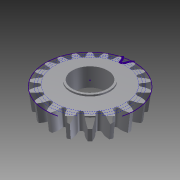
# Autodesk Inventor part: Z20
Saved by Autodesk Inventor 2014 (Build 180170000, 170)
## iProperties
Created: 2013-05-24
Part Number: Z20
Material: Generic
Document SubType Name: Modeling
Designer: hartmann
Density: 1 g/cm^3
Appearance: Default
Mass: 0.0697017 g
Surface Area: 1.89234 cm^2
Volume: 0.0697017 cm^3
Author: hartmann
Autodesk Inventor part; units mm, degrees
ref_plane "YZ Plane" through (0, 0, 0) normal (1, 0, 0) x (0, 1, 0)
ref_plane "XZ Plane" through (0, 0, 0) normal (0, 1, 0) x (-1, 0, 0)
ref_plane "XY Plane" through (0, 0, 0) normal (0, 0, 1) x (1, 0, 0)
sketch "Sketch1" plane through (0, 0, 0) normal (0, 0, 1) x (1, 0, 0)
  spline S0 degree 3 poles (-0.5498, 4.3643) (-0.5222, 4.3285) (-0.4672, 4.2569) (-0.3937, 4.1428) (-0.3394, 4.0438) (-0.3016, 3.9617) (-0.2765, 3.8987) (-0.2553, 3.8344) (-0.2398, 3.7683) (-0.2337, 3.7121) (-0.2228, 3.6682) (-0.211, 3.6364) (-0.1968, 3.6056) (-0.1785, 3.577) (-0.156, 3.5515) (-0.13, 3.5296) (-0.1002, 3.5131) (-0.0677, 3.503) (-0.0339, 3.4991) (0, 3.5004) (0.0339, 3.4991) (0.0677, 3.503) (0.1002, 3.5131) (0.13, 3.5296) (0.156, 3.5515) (0.1785, 3.577) (0.1968, 3.6056) (0.211, 3.6364) (0.2228, 3.6682) (0.2337, 3.7121) (0.2398, 3.7683) (0.2553, 3.8344) (0.2765, 3.8987) (0.3016, 3.9617) (0.3394, 4.0438) (0.3937, 4.1428) (0.4672, 4.2569) (0.5222, 4.3285) (0.5498, 4.3643) knots 0 0 0 0 0.062514 0.125029 0.187537 0.218798 0.250057 0.281314 0.31256 0.343809 0.359439 0.375065 0.39068 0.406298 0.421914 0.437531 0.453156 0.468766 0.484369 0.5 0.515631 0.531234 0.546844 0.562469 0.578086 0.593702 0.60932 0.624935 0.640561 0.656191 0.68744 0.718686 0.749943 0.781202 0.812463 0.874971 0.937486 1 1 1 1
  circle A0 centre (0, 0) radius 3.5 construction
  circle A1 centre (0, 0) radius 3.7588 construction
  circle A2 centre (0, 0) radius 4 construction
  circle A3 centre (0, 0) radius 4.3988
  point P0 (-0.4687, 4.2558)
  point P1 (-0.3951, 4.142)
  point P2 (-0.3304, 4.023)
  point P3 (-0.3021, 3.9615)
  point P4 (-0.2771, 3.8985)
  point P5 (-0.2562, 3.8341)
  point P6 (-0.2412, 3.7681)
  point P7 (-0.2305, 3.7012)
  point P8 (-0.2222, 3.6683)
  point P9 (-0.2106, 3.6365)
  point P10 (-0.1961, 3.606)
  point P11 (-0.1778, 3.5775)
  point P12 (-0.1554, 3.5521)
  point P13 (-0.1294, 3.5305)
  point P14 (-0.0997, 3.5142)
  point P15 (-0.0674, 3.504)
  point P16 (-0.0339, 3.5)
  point P17 (0, 3.5)
  point P18 (0.0339, 3.5)
  point P19 (0.0674, 3.504)
  point P20 (0.0997, 3.5142)
  point P21 (0.1294, 3.5305)
  point P22 (0.1554, 3.5521)
  point P23 (0.1778, 3.5775)
  point P24 (0.1961, 3.606)
  point P25 (0.2106, 3.6365)
  point P26 (0.2222, 3.6683)
  point P27 (0.2305, 3.7012)
  point P28 (0.2412, 3.7681)
  point P29 (0.2562, 3.8341)
  point P30 (0.2771, 3.8985)
  point P31 (0.3021, 3.9615)
  point P32 (0.3304, 4.023)
  point P33 (0.3951, 4.142)
  point P34 (0.4687, 4.2558)
  constraints: 4 centre point, 2 point on circle, 79 other
extrude "Extrusion1" add sketch "Sketch1" against normal blind 1.7
extrude "Extrusion2" cut sketch "Sketch1" against normal through all contours A3 S0 picked at (0.0657, 4.1822)
pattern_circular "Runde Anordnung1" count 20 over 360 about axis through (0, 0, -10) along (0, 0, 1) of "Extrusion2"
sketch "Sketch4" plane through (0, 0, 0) normal (0, 0, 1) x (1, 0, 0)
  circle A0 centre (0, 0) radius 1.75
  circle A1 centre (0, 0) radius 1.75
  constraints: 2 centre point, 1 coincident, 1 concentric, 2 other
extrude "Extrusion5" cut sketch "Sketch4" against normal through all
sketch "Sketch5" plane through (0, 0, -1.7) normal (0, 0, -1) x (-1, 0, 0)
  circle A0 centre (0, 0) radius 1.75 projected
  arc A1 (-0.5498, 4.3643) -> (-0.8258, 4.3206) centre (0, 0) ccw projected
  circle A2 centre (0, 0) radius 2.25
  dimension "d14" = 0.5
  constraints: 1 centre point, 1 coincident
  measures "d14" radial gap between concentric circles of A2 A0
extrude "Extrusion6" add sketch "Sketch5" along normal blind 0.15
sketch "Sketch6" plane through (0, 0, 0) normal (0, 0, 1) x (1, 0, 0)
  circle A0 centre (0, 0) radius 1.75 projected
  circle A1 centre (0, 0) radius 2.25 projected
extrude "Extrusion7" add sketch "Sketch6" along normal blind 0.15
equation "\"Modul\" = 0.4"
equation "\"Druckwinkel\" = 20deg"
equation "\"UnitProfileClearance\" = 0.25"
equation "\"UnitRoundRadius\" = 0.35"
equation "\"Kopfdurchmesser\" = 8.79756"
equation "\"Stammdurchmesser\" = 7"
equation "\"Grundkreisdurchmesser\" = 7.51754"
equation "\"Gewindedurchmesser\" = 8"
equation "\"Zahnbreite\" = 2"
equation "\"Schrägungswinkel\" = 0"
equation "\"UnitCorrection\" = 0"
equation "\"UnitAddendumModification\" = 0.003054"
equation "\"Zahnkreisteilung\" = 1.25664"
equation "\"UnitBacklashShift\" = 0"
equation "\"Gesamtzahnstärke\" = 0"
equation "\"Innen\" = 0"
